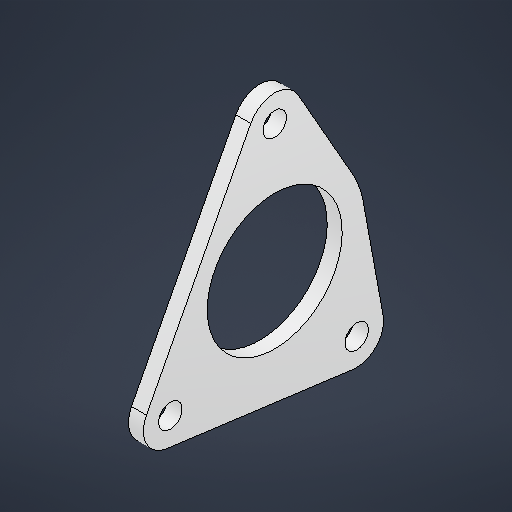
# Autodesk Inventor part: PLATE,REVERSER,SUPPORT
Saved by Autodesk Inventor 2026.1 (Build 301233020, 233B)
## iProperties
Created: 2026-02-14
Part Number: PLATE,REVERSER,SUPPORT
Material: Aluminum 6061
Document SubType Name: Sheet Metal
Designer: Owen L
Density: 2.7 g/cm^3
Sheet Metal Rule: Default
Appearance: Aluminum - Flat
Author: Owen L
Autodesk Inventor part; units mm, degrees
ref_plane "YZ Plane" through (0, 0, 0) normal (1, 0, 0) x (0, 1, 0)
ref_plane "XZ Plane" through (0, 0, 0) normal (0, 1, 0) x (-1, 0, 0)
ref_plane "XY Plane" through (0, 0, 0) normal (0, 0, 1) x (1, 0, 0)
sketch "Sketch1" plane through (0, 0, 0) normal (1, 0, 0) x (0, 1, 0)
  line L0 (-15.4794, 22.1069) -> (0, 0) construction
  line L1 (0, 0) -> (26.9875, 0) construction
  line L2 (0, 0) -> (-20.6736, -17.3472) construction
  arc A0 (-12.8405, 27.1761) -> (-21.1455, 22.8528) centre (-15.4794, 22.1069) ccw
  arc A1 (-26.3397, -16.6013) -> (-19.6431, -22.9686) centre (-20.6736, -17.3472) ccw
  arc A2 (29.8114, -4.9686) -> (29.6264, 5.0693) centre (26.9875, 0) ccw
  circle A3 centre (0, 0) radius 14.2875 construction
  line L3 (9.4129, -16.562) -> (29.8114, -4.9686)
  arc A4 (3.4351, -18.7377) -> (9.4129, -16.562) centre (0, 0) ccw
  line L4 (3.4351, -18.7377) -> (-19.6431, -22.9686)
  line L5 (-26.3397, -16.6013) -> (-21.1455, 22.8528)
  line L6 (-12.8405, 27.1761) -> (29.6264, 5.0693)
  line L7 (0, 0) -> (0, -5.4993)
  dimension "d0" = 26.9875
  dimension "d1" = 95
  dimension "d2" = 5.715
  dimension "d3" = 28.575
  dimension "d22" = 19.05
  dimension "d23" = 50
  constraints: 16 end point, 8 point on circle, 8 tangent, 6 coincident, 5 centre point, 2 equal length, 2 equal radius, 1 horizontal, 1 horizontal alignment, 1 vertical
  measures "d0" distance of point (0, 0) L1.end
  measures "d1" angle of L0 L2
  measures "d2" radius of A0
  measures "d3" diameter of A3
  measures "d22" radius of A4
  measures "d23" angle of L2 L7
extrude "Plate1" add sketch "Sketch1" along normal blind 3.175
hole "Hole1" at (0, 0, 0) direction (1, 0, 0) diameter 28.575 depth 3.175 tip angle 118
hole "Hole2" at (0, 26.9875, 0) at (0, -15.4794, 22.1069) at (0, -20.6736, -17.3472) direction (1, 0, 0) diameter 4.9784 depth 3.175 tip angle 118 clearance for "Flat Head Machine Screw (82)" size "#10" standard "Ansi Unified Screw Threads"
equation "\"d11\" = Thickness"
equation "\"d18\" = Thickness"
equation "\"d5\" = Thickness"
equation "\"BendRadius\" = Thickness"
equation "\"BendReliefWidth\" = Thickness"
equation "\"BendReliefDepth\" = 0.5 * Thickness"
equation "\"CornerReliefSize\" = 4 * Thickness"
equation "\"MinimumRemnant\" = 2 * Thickness"
equation "\"TransitionRadius\" = BendRadius"
equation "\"JacobiRadiusSize\" = BendRadius"
equation "\"GapSize\" = Thickness"
equation "\"Thickness\" = 3.175"
body "Solid1"
